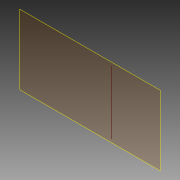
# Autodesk Inventor part: RedLine
Saved by Autodesk Inventor 2013 (Build 170138000, 138)
## iProperties
Created: 2013-01-07
Part Number: RedLine
Material: ABS Plastic
Document SubType Name: Modeling
Designer: Phillip
Density: 1 g/cm^3
Author: Phillip
Autodesk Inventor part; units mm, degrees
ref_plane "YZ Plane" through (0, 0, 0) normal (1, 0, 0) x (0, 1, 0)
ref_plane "XZ Plane" through (0, 0, 0) normal (0, 1, 0) x (-1, 0, 0)
ref_plane "XY Plane" through (0, 0, 0) normal (0, 0, 1) x (1, 0, 0)
ref_plane "Work Plane1" through (0, 0, 0) normal (0, 0, 1) x (1, 0, 0)
sketch "Sketch1" plane through (0, 0, 0) normal (0, 0, 1) x (1, 0, 0)
  line L0 (-8248.396, -4082.669) -> (8248.396, -4082.669) projected
  line L1 (8248.396, -4082.669) -> (8248.396, 4082.669) projected
  line L2 (8248.396, 4082.669) -> (-8248.396, 4082.669) projected
  line L3 (-8248.396, 4082.669) -> (-8248.396, -4082.669) projected
  line L4 (2716.7308, 4082.669) -> (2767.5308, 4082.669)
  line L5 (2767.5308, 4082.669) -> (2767.5308, -4082.669)
  line L6 (2767.5308, -4082.669) -> (2716.7308, -4082.669)
  line L7 (2716.7308, -4082.669) -> (2716.7308, 4082.669)
  line L8 (-8248.396, -4082.669) -> (8248.396, -4082.669) projected
  line L9 (8248.396, -4082.669) -> (8248.396, 4082.669) projected
  line L10 (8248.396, 4082.669) -> (-8248.396, 4082.669) projected
  line L11 (-8248.396, 4082.669) -> (-8248.396, -4082.669) projected
  line L12 (2743.2, -7112) -> (2743.2, 7112)
  point P0 (0, 0)
  point P1 (2742.1308, 4082.669)
  dimension "d0" = 50.8
  constraints: 10 end point, 2 collinear, 2 parallel, 1 horizontal, 1 midpoint, 1 perpendicular, 1 vertical, 2 other
  measures "d0" distance of L4.start L4.end
extrude "Extrusion1" add sketch "Sketch1" along normal blind 2.54 contours L7 L2 L12 L0 | L12 L2 L5 L0
body "Solid1"
